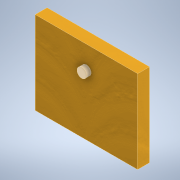
# Autodesk Inventor part: SensorSupport
Saved by Autodesk Inventor 2022.2 (Build 262287010, 287A)
## iProperties
Created: 2022-05-29
Part Number: SensorSupport
Material: Plástico ABS
Document SubType Name: Modeling
Designer: mabel
Density: 1.06 g/cm^3
Appearance: Soldadura - Latón
Author: mabel
Autodesk Inventor part; units mm, degrees
ref_plane "YZ Plane" through (0, 0, 0) normal (1, 0, 0) x (0, 1, 0)
ref_plane "XZ Plane" through (0, 0, 0) normal (0, 1, 0) x (-1, 0, 0)
ref_plane "XY Plane" through (0, 0, 0) normal (0, 0, 1) x (1, 0, 0)
sketch "Boceto1" plane through (0, 0, 0) normal (0, 0, 1) x (1, 0, 0)
  line L0 (21.572, -17.5) -> (-21.572, -17.5)
  line L1 (-21.572, -17.5) -> (-21.572, 17.5)
  line L2 (-21.572, 17.5) -> (21.572, 17.5)
  line L3 (21.572, 17.5) -> (21.572, -17.5)
  line L4 (21.572, -17.5) -> (-21.572, 17.5) construction
  line L5 (-21.572, -17.5) -> (21.572, 17.5) construction
  circle A0 centre (0, 8) radius 1.75
  point P0 (0, 0)
  dimension "d0" = 43.144
  dimension "d1" = 35
  dimension "d3" = 3.5
  constraints: 12 end point, 2 midpoint, 2 parallel, 1 centre point, 1 horizontal, 1 perpendicular
  measures "d0" distance of L1.end L2.end
  measures "d1" distance of L0.end L1.end
  measures "d3" diameter of A0
extrude "Extrusión1" add sketch "Boceto1" along normal blind 5
sketch "Boceto3" plane through (0, 0, 5) normal (0, 0, 1) x (1, 0, 0)
  circle A0 centre (0, 8) radius 1.75 projected
  circle A1 centre (0, 8) radius 2
  point P0 (0, 0)
  dimension "d6" = 4
  constraints: 1 centre point, 1 coincident
  measures "d6" diameter of A1
extrude "Extrusión2" add sketch "Boceto3" along normal blind 2 contours A0 | A1
